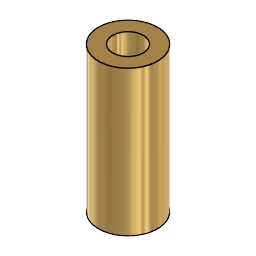
Mp3 PCB CAD Assembly (Autodesk Fusion 360 archive; units mm, degrees)
design "brass 10mm standoffs"
part number: 2026-06-01-13-56-33-233
Autodesk Fusion 360 part; units mm, degrees
sketch "Sketch1" plane through (0, 0, 0) normal (0, 0, 1) x (1, 0, 0)
  circle A0 centre (0, 0) radius 1.05
  circle A1 centre (0, 0) radius 2.032
  dimension "d1" = 2.1
  constraint coincident A0.centre A1.centre
  measures "d1" diameter of A0
extrude "Extrude1" add sketch "Sketch1" along normal blind 10
